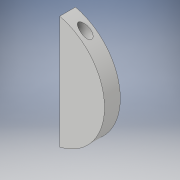
# Autodesk Inventor part: Contrapeso4
Saved by Autodesk Inventor 2019 (Build 230136000, 136)
## iProperties
Created: 2019-06-29
Part Number: Contrapeso4
Material: Generic
Document SubType Name: Modeling
Designer: usuario
Density: 1 g/cm^3
Appearance: Default
Mass: 6.18429 g
Surface Area: 27.9901 cm^2
Volume: 6.18429 cm^3
Author: usuario
Autodesk Inventor part; units mm, degrees
ref_plane "YZ Plane" through (0, 0, 0) normal (1, 0, 0) x (0, 1, 0)
ref_plane "XZ Plane" through (0, 0, 0) normal (0, 1, 0) x (-1, 0, 0)
ref_plane "XY Plane" through (0, 0, 0) normal (0, 0, 1) x (1, 0, 0)
sketch "Sketch1" plane through (0, 0, 0) normal (0, 0, 1) x (1, 0, 0)
  line L0 (6.2115, -26.7893) -> (6.2115, 26.924)
  line L1 (6.2115, 26.7893) -> (6.2115, -26.7893)
  arc A0 (6.2115, -26.924) -> (6.2115, 26.924) centre (-0.1699, 0) ccw
  line L2 (6.2115, 26.924) -> (6.2115, -26.924)
  point P0 (0, 0)
  point P1 (-5.2115, 24.6247)
  constraints: 6 end point, 2 point on circle, 2 point on line, 1 centre point, 1 collinear
extrude "Extrusion1" add sketch "Sketch1" along normal blind 7.5
sketch "Sketch2" plane through (6.2115, -26.924, 0) normal (-1, 0, 0) x (0, 0, 1)
  line L0 (0, 6.9167) -> (7.5, 6.9167)
  line L1 (0, 0) -> (0, 6.9167)
  line L2 (0, 6.9167) -> (7.5, 6.9167)
  line L3 (7.5, 26.7893) -> (7.5, 0)
  line L4 (7.5, 6.9167) -> (7.5, 0)
  line L5 (7.5, 0) -> (0, 0)
  line L6 (7.5, 0) -> (0, 0)
  circle A0 centre (3.75, 3.4583) radius 1
  line L7 (0, 0) -> (0, 53.5786)
  line L8 (0, 53.5786) -> (0, 0)
  line L9 (0, 26.7893) -> (7.5, 26.7893)
  circle A1 centre (3.75, 50.1203) radius 1
  circle A2 centre (3.75, 3.4583) radius 2
  circle A3 centre (3.75, 50.1203) radius 2
  point P0 (0, 26.924)
  point P1 (280.32, 51.414)
  point P2 (4.4851, 4.1363)
  point P3 (4.4851, 2.7804)
  point P4 (3.0149, 4.1363)
  point P5 (3.0149, 2.7804)
  dimension "d2" = 2
  dimension "d5" = 4
  dimension "d6" = 4
  constraints: 20 end point, 4 centre point, 4 point on circle, 2 coincident, 2 perpendicular, 2 vertical, 1 collinear, 1 midpoint, 1 symmetric about line, 1 other
  measures "d2" diameter of A0
  measures "d5" diameter of A2
  measures "d6" diameter of A3
extrude "Extrusion2" cut sketch "Sketch2" against normal blind 25.4 contours A0 | A1
extrude "Extrusion3" cut sketch "Sketch2" against normal blind 16.35 contours A2 | A3
scale "Scale1" factors (0.5, 0.5, 0.5) then translate (3.1057, 0, 3.75) bodies 1
body "Solid1"
